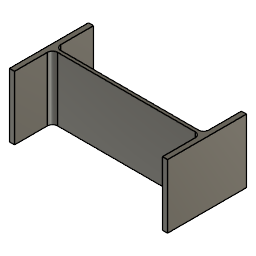
H-248×124×5×8 (Autodesk Fusion 360 design; units mm, degrees)
Autodesk Fusion 360 part; units mm, degrees
sketch "スケッチ1" plane through (0, 0, 0) normal (0, 0, 1) x (1, 0, 0)
  line L0 (232, 2.5) -> (16, 2.5)
  line L1 (16, -2.5) -> (232, -2.5)
  line L2 (0, 62) -> (0, -62)
  line L3 (8, 10.5) -> (8, 62)
  line L4 (8, -62) -> (8, -10.5)
  line L5 (0, -62) -> (8, -62)
  line L6 (8, 62) -> (0, 62)
  line L7 (240, 62) -> (240, 10.5)
  line L8 (248, -62) -> (248, 62)
  line L9 (240, -10.5) -> (240, -62)
  line L10 (240, -62) -> (248, -62)
  line L11 (248, 62) -> (240, 62)
  arc A0 (16, -2.5) -> (8, -10.5) centre (16, -10.5) ccw
  arc A1 (8, 10.5) -> (16, 2.5) centre (16, 10.5) ccw
  arc A2 (232, 2.5) -> (240, 10.5) centre (232, 10.5) ccw
  arc A3 (240, -10.5) -> (232, -2.5) centre (232, -10.5) ccw
extrude "押し出し1" add sketch "スケッチ1" along normal blind 100
